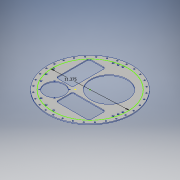
# Autodesk Inventor part: mini 55K stage
Saved by Autodesk Inventor 2018 (Build 220112000, 112)
## iProperties
Created: 2018-10-16
Part Number: mini 55K stage
Material: Aluminum 6061
Document SubType Name: Modeling
Designer: freyja
Density: 2.7 g/cm^3
Appearance: Aluminum - Flat
Mass: 408.876 g
Surface Area: 1052.96 cm^2
Volume: 151.436 cm^3
Author: freyja
Autodesk Inventor part; units mm, degrees
ref_plane "YZ Plane" through (0, 0, 0) normal (1, 0, 0) x (0, 1, 0)
ref_plane "XZ Plane" through (0, 0, 0) normal (0, 1, 0) x (-1, 0, 0)
ref_plane "XY Plane" through (0, 0, 0) normal (0, 0, 1) x (1, 0, 0)
sketch "Sketch2" plane through (0, 0, 0) normal (0, 1, 0) x (-1, 0, 0)
  line L0 (0, 0) -> (-28.0184, -28.0184) construction
  line L1 (0, 0) -> (-39.624, 0) construction
  circle A0 centre (-28.0184, -28.0184) radius 161.925
  dimension "d6" = 39.624
  dimension "d7" = 315
  dimension "d8" = 323.85
  constraints: 4 end point, 1 centre point, 1 coincident, 1 equal length, 1 horizontal
  measures "d6" distance of L0.start L0.end
  measures "d8" diameter of A0
extrude "Extrusion1" add sketch "Sketch2" against normal blind 3.175
sketch "Sketch1" plane through (0, 0, 0) normal (0, 1, 0) x (-1, 0, 0)
  line L0 (0, 0) -> (-64.6578, -64.6578) construction
  line L1 (0, 0) -> (91.44, 0) construction
  circle A0 centre (-64.6578, -64.6578) radius 69.85
  line L2 (0, 0) -> (40.4112, 40.4112) construction
  line L3 (0, 0) -> (57.15, 0) construction
  circle A1 centre (40.4112, 40.4112) radius 38.1
  dimension "d0" = 91.44
  dimension "d1" = 135
  dimension "d2" = 139.7
  dimension "d3" = 57.15
  dimension "d4" = 45
  dimension "d5" = 76.2
  constraints: 8 end point, 2 centre point, 2 coincident, 2 equal length, 2 horizontal
  measures "d0" distance of L0.start L0.end
  measures "d1" angle of L0 L1
  measures "d2" diameter of A0
  measures "d3" distance of L0.start L2.end
  measures "d4" angle of L3 L2
  measures "d5" diameter of A1
extrude "Extrusion2" cut sketch "Sketch1" against normal up to surface (3.175 mm away)
sketch "Sketch6" plane through (28.0184, 0, -28.0184) normal (0, 1, 0) x (1, 0, 0)
  circle A0 centre (0, 0) radius 161.925 projected
  line L0 (0, 0) -> (154.3504, 13.5039)
  line L1 (0, 0) -> (154.94, 0) construction
  point P0 (-28.0184, -28.0184)
  dimension "d65" = 154.94
  dimension "d66" = 5
  constraints: 4 end point, 1 equal length, 1 horizontal
  measures "d65" distance of L0.start L0.end
  measures "d66" angle of L1 L0
hole "Hole3" at (182.3688, 0, -41.5223) direction (0, -1, 0) diameter 4.9784 end through all thread size "1/4-20 UNC" class "2B" standard "ANSI Unified Screw Threads"
pattern_circular "Circular Pattern1" count 32 over 360 about axis through (28.0184, 0, -28.0184) along (0, -1, 0) of "Hole3"
sketch "Sketch11" plane through (28.0184, 0, -28.0184) normal (0, 1, 0) x (1, 0, 0)
  line L0 (-28.0184, -28.0184) -> (137.3706, 110.7594) construction
  line L1 (-28.0184, -28.0184) -> (187.8816, -28.0184) construction
  line L2 (-28.0184, -28.0184) -> (110.7594, 137.3706) construction
  line L3 (-28.0184, -28.0184) -> (187.8816, -28.0184) construction
  circle A0 centre (137.3706, 110.7594) radius 123.2917
  circle A1 centre (110.7594, 137.3706) radius 123.2917
  circle A2 centre (-166.7962, 137.3706) radius 123.2917
  circle A3 centre (-193.4074, 110.7594) radius 123.2917
  circle A4 centre (-193.4074, -166.7962) radius 123.2917
  circle A5 centre (-166.7962, -193.4074) radius 123.2917
  circle A6 centre (110.7594, -193.4074) radius 123.2917
  circle A7 centre (137.3706, -166.7962) radius 123.2917
  line L4 (0, 0) -> (196.85, 0) construction
  circle A8 centre (0, 0) radius 161.925 projected
  line L5 (0, 0) -> (-150.7958, -126.5327)
  line L6 (0, 0) -> (196.85, 0) construction
  line L7 (0, 0) -> (-126.5327, -150.7958)
  line L8 (0, 0) -> (196.85, 0) construction
  circle A9 centre (-150.7958, -126.5327) radius 123.2917 construction
  circle A10 centre (-126.5327, -150.7958) radius 123.2917 construction
  circle A11 centre (0, 0) radius 139.7
  point P0 (138.6284, 17.2699)
  point P1 (132.7246, -43.5921)
  point P2 (-0.2196, -139.6998)
  point P3 (-139.6998, -0.2196)
  point P4 (-43.5921, 132.7246)
  point P5 (-12.5196, 139.1379)
  point P6 (139.1379, -12.5196)
  point P7 (-65.2058, -123.5488)
  point P8 (-123.5488, -65.2058)
  dimension "d101" = 246.5835
  dimension "d147" = 279.4
  dimension "d97" = 215.9
  dimension "d98" = 40
  dimension "d99" = 215.9
  dimension "d100" = 50
  dimension "d102" = 246.5835
  dimension "d105" = 360
  dimension "d109" = 196.85
  dimension "d110" = 140
  dimension "d111" = 196.85
  dimension "d112" = 130
  dimension "d148" = 246.5835
  dimension "d149" = 246.5835
  constraints: 18 end point, 5 coincident, 5 horizontal, 4 equal length, 3 centre point, 2 point on circle, 49 other
  measures "d97" distance of L0.start L0.end
  measures "d98" angle of L1 L0
  measures "d99" distance of L0.start L2.end
  measures "d100" angle of L3 L2
  measures "d102" diameter of A1
  measures "d109" distance of L5.start L5.end
  measures "d110" angle of L5 L6
  measures "d111" distance of L5.start L7.end
  measures "d112" angle of L7 L8
  measures "d148" diameter of A9
  measures "d149" diameter of A10
hole "Hole5" at (-111.6814, 0, -27.7988) at (160.743, 0, 15.5737) at (-15.5737, 0, -160.743) at (15.4988, 0, -167.1563) at (167.1563, 0, -15.4988) at (27.7988, 0, 111.6814) at (-95.5304, 0, 37.1874) at (-37.1874, 0, 95.5304) direction (0, -1, 0) diameter 6.7564 end through all clearance for "Flat Head Machine Screw (82)" size "1/4" standard "Ansi Unified Screw Threads"
sketch "Sketch12" plane through (28.0184, 0, -28.0184) normal (0, 1, 0) x (1, 0, 0)
  circle A0 centre (0, 0) radius 161.925 projected
  line L0 (-28.0184, -28.0184) -> (6.2716, -28.0184) construction
  line L1 (0, 0) -> (-28.2385, 136.8162)
  line L2 (0, 0) -> (139.7, 0) construction
  circle A1 centre (-43.5921, 132.7246) radius 3.3782 projected
  circle A2 centre (-12.5196, 139.1379) radius 3.3782 projected
  line L3 (-43.5921, 132.7246) -> (-12.5196, 139.1379)
  circle A3 centre (132.7246, -43.5921) radius 3.3782 projected
  circle A4 centre (139.1379, -12.5196) radius 3.3782 projected
  line L4 (132.7246, -43.5921) -> (139.1379, -12.5196)
  line L5 (0, 0) -> (136.8162, -28.2385)
  line L6 (0, 0) -> (-135.5756, -33.6947)
  circle A5 centre (-139.6998, -0.2196) radius 3.3782 projected
  circle A6 centre (-123.5488, -65.2058) radius 3.3782 projected
  line L7 (-139.6998, -0.2196) -> (-123.5488, -65.2058)
  circle A7 centre (-65.2058, -123.5488) radius 3.3782 projected
  circle A8 centre (-0.2196, -139.6998) radius 3.3782 projected
  line L8 (-65.2058, -123.5488) -> (-0.2196, -139.6998)
  line L9 (0, 0) -> (-33.6947, -135.5756)
  point P0 (136.8162, -28.2385)
  point P1 (-33.6947, -135.5756)
  dimension "d150" = 139.7
  dimension "d152" = 139.7
  dimension "d153" = 139.7
  dimension "d154" = 139.7
  constraints: 20 end point, 4 coincident, 4 perpendicular, 2 horizontal, 1 equal length
  measures "d150" distance of L1.start L1.end
  measures "d152" distance of L1.start L5.end
  measures "d153" distance of L1.start L6.end
  measures "d154" distance of L1.start L9.end
hole "Hole6" at (-0.2201, 0, -164.8346) at (-107.5572, 0, 5.6763) at (-5.6763, 0, 107.5572) at (164.8346, 0, 0.2201) direction (0, -1, 0) diameter 6.7564 end through all clearance for "Flat Head Machine Screw (82)" size "1/4" standard "Ansi Unified Screw Threads"
sketch "Sketch13" plane through (28.0184, 0, -28.0184) normal (0, 1, 0) x (1, 0, 0)
  line L0 (-41.91, -25.4) -> (-41.91, 101.6)
  line L1 (-41.91, 101.6) -> (-105.41, 101.6)
  line L2 (-105.41, 101.6) -> (-105.41, -25.4)
  line L3 (-105.41, -25.4) -> (-41.91, -25.4)
  line L4 (-41.91, -25.4) -> (-105.41, 101.6) construction
  line L5 (-41.91, 101.6) -> (-105.41, -25.4) construction
  line L6 (-41.91, -25.4) -> (85.09, -25.4) construction
  circle A0 centre (0, 0) radius 161.925 projected
  line L7 (0, 0) -> (17.9605, 17.9605)
  line L8 (0, 0) -> (25.4, 0) construction
  line L9 (-25.4, -41.91) -> (101.6, -41.91)
  line L10 (101.6, -41.91) -> (101.6, -105.41)
  line L11 (101.6, -105.41) -> (-25.4, -105.41)
  line L12 (-25.4, -105.41) -> (-25.4, -41.91)
  line L13 (0, 0) -> (-73.66, 0) construction
  line L14 (0, 0) -> (73.66, 0) construction
  line L15 (-73.66, 0) -> (-73.66, 38.1) construction
  point P0 (-28.0184, -28.0184)
  dimension "d155" = 127
  dimension "d156" = 90
  dimension "d157" = 63.5
  dimension "d160" = 25.4
  dimension "d161" = 45
  dimension "d164" = 73.66
  dimension "d165" = 180
  dimension "d166" = 38.1
  dimension "d167" = 90
  constraints: 32 end point, 4 horizontal, 4 symmetric about line, 3 equal length, 2 parallel, 2 perpendicular, 1 midpoint
  measures "d155" distance of L0.start L0.end
  measures "d156" angle of L6 L0
  measures "d157" distance of L0.end L1.end
  measures "d160" distance of L7.start L7.end
  measures "d161" angle of L8 L7
  measures "d164" distance of L7.start L13.end
  measures "d165" angle of L13 L14
  measures "d166" distance of L15.end L13.end
  measures "d167" angle of L13 L15
extrude "Extrusion3" cut sketch "Sketch13" against normal blind 25.4 contours L3 L2 L1 L0 | L9 L10 L11 L12
fillet "Fillet1" radius 6.35 8 edges at (-13.8916, -1.5875, -129.6184) (-77.3916, -1.5875, -129.6184) (-77.3916, -1.5875, -2.6184) (-13.8916, -1.5875, -2.6184) (129.6184, -1.5875, 77.3916) (2.6184, -1.5875, 13.8916) (2.6184, -1.5875, 77.3916) (129.6184, -1.5875, 13.8916)
sketch "Sketch14" plane through (28.0184, 0, -28.0184) normal (0, 1, 0) x (1, 0, 0)
  line L0 (-97.6396, -97.6396) -> (-39.2196, -97.6396) construction
  line L1 (-39.2196, -97.6396) -> (-39.2196, -39.2196) construction
  line L2 (-39.2196, -39.2196) -> (-97.6396, -39.2196) construction
  line L3 (-97.6396, -39.2196) -> (-97.6396, -97.6396) construction
  circle A0 centre (-68.4296, -68.4296) radius 38.1 projected
  line L4 (-97.6396, -97.6396) -> (-39.2196, -39.2196) construction
  line L5 (-39.2196, -97.6396) -> (-97.6396, -39.2196) construction
  point P0 (-28.0184, -28.0184)
  dimension "d169" = 58.42
  dimension "d170" = 58.42
  constraints: 12 end point, 4 coincident, 2 midpoint, 2 parallel, 1 horizontal, 1 perpendicular
  measures "d169" distance of L2.end L1.end
  measures "d170" distance of L1.end L0.end
sketch "Sketch15" plane through (28.0184, 0, -28.0184) normal (0, 1, 0) x (1, 0, 0)
  circle A0 centre (0, 0) radius 144.4625
  point P0 (-28.0184, -28.0184)
  dimension "d171" = 288.925
  constraints: 1 centre point
  measures "d171" diameter of A0
hole "Hole7" at (-11.2012, 0, 11.2012) at (-11.2012, 0, 69.6212) at (-69.6212, 0, 69.6212) at (-69.6212, 0, 11.2012) direction (0, -1, 0) diameter 4.4958 end through all clearance for "Flat Head Machine Screw (82)" size "#8" standard "Ansi Unified Screw Threads"
equation "\"d101\" = d102"
equation "\"d148\" = d102"
equation "\"d149\" = d102"
body "Solid1"
